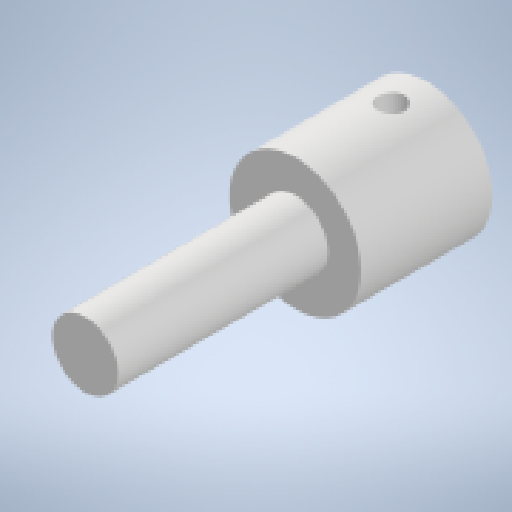
# Autodesk Inventor part: acoplador sensor
Saved by Autodesk Inventor 2023 (Build 270158000, 158)
## iProperties
Created: 2022-10-25
Part Number: acoplador sensor
Material: Generic
Document SubType Name: Modeling
Designer: klebe
Density: 1 g/cm^3
Appearance: Default
Author: klebe
Autodesk Inventor part; units mm, degrees
ref_plane "YZ Plane" through (0, 0, 0) normal (1, 0, 0) x (0, 1, 0)
ref_plane "XY Plane" through (0, 0, 0) normal (0, 0, 1) x (1, 0, 0)
sketch "Sketch1" plane through (0, 0, 0) normal (0, 0, 1) x (1, 0, 0)
  circle A0 centre (25, 22.275) radius 1 projected
  circle A1 centre (25, 22.275) radius 5
  circle A2 centre (25, 22.275) radius 1
  point P0 (0, 0)
  dimension "d0" = 10
  dimension "d6" = 2
  constraints: 2 centre point, 1 coincident
  measures "d0" diameter of A1
  measures "d6" diameter of A2
extrude "Extrusion1" add sketch "Sketch1" along normal blind 30
sketch "Sketch2" plane through (25, 22.275, 30) normal (0, 0, 1) x (1, 0, 0)
  circle A0 centre (0, 0) radius 5 projected
  circle A1 centre (0, 0) radius 2.5
  circle A2 centre (0, 0) radius 1
  point P0 (-25, -22.275)
  constraints: 2 centre point, 1 coincident
extrude "Extrusion2" add sketch "Sketch2" along normal blind 16 contours A1
ref_plane "Work Plane1" through (25, 27.275, 0) normal (0, 1, 0) x (-1, 0, 0)
sketch "Sketch4" plane through (25, 27.275, 0) normal (0, 1, 0) x (-1, 0, 0)
  circle A0 centre (0, 5) radius 1
  line L0 (5, 30) -> (-5, 30) projected
  line L1 (5, 0) -> (-5, 0) projected
  line L2 (5, 30) -> (-5, 30) projected
  line L3 (0, 30) -> (5, 30)
  line L4 (0, 30) -> (0, 25)
  point P0 (25, 0)
  dimension "d8" = 2
  dimension "d18" = 5
  dimension "d19" = 5
  constraints: 4 end point, 1 centre point, 1 midpoint, 1 vertical
  measures "d8" diameter of A0
  measures "d18" distance of L3.start L0.start
  measures "d19" distance of L3.start L4.end
hole "Hole1" at (25, 27.275, 5) direction (0, -1, 0) diameter 2.2 depth 5 tip angle 118
sketch "Sketch5" plane through (25, 22.275, 46) normal (0, 0, 1) x (1, 0, 0)
  circle A0 centre (0, 0) radius 1
  point P0 (-25, -22.275)
  constraints: 1 centre point
extrude "Extrusion3" add sketch "Sketch5" against normal blind 36
body "Solid1"
